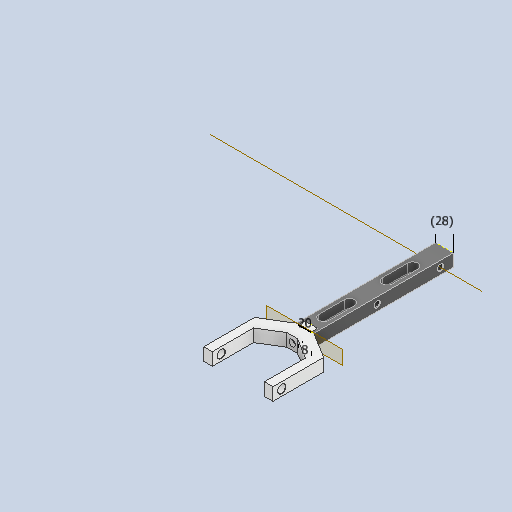
# Autodesk Inventor part: Adaptationhorizontalachse_Rillenkugellager
Saved by Autodesk Inventor 2024 (Build 280153000, 153)
## iProperties
Created: 2022-02-28
Part Number: Adaptationhorizontalachse_Rillenkugellager
Material: PBT-Kunststoff
Document SubType Name: Modeling
Designer: 123St
Density: 1.31 g/cm^3
Appearance: Glatt - Weiß
Mass: 228.778 g
Surface Area: 480.28 cm^2
Volume: 174.64 cm^3
Fixation_dist1: -20,000 mm
Fixation_dist2: -100,000 mm
Gabel_FixierungPart_Width: 28,000 mm
Author: 123St
Autodesk Inventor part; units mm, degrees
note: some values were not read from the file. Chosen so that the rebuilt part matches the saved one: direction of "Bohrung3"; direction of "Bohrung4".
sketch "Skizze1" plane through (0, 0, 0) normal (0, 1, 0) x (-1, 0, 0)
  line L0 (54.5, 104.8161) -> (54.5, 24.8161)
  line L1 (54.5, 24.8161) -> (14, 0)
  line L2 (14, 0) -> (-14, 0)
  line L3 (-14, 0) -> (-54.5, 24.8161)
  line L4 (-54.5, 24.8161) -> (-54.5, 104.8161)
  line L5 (-54.5, 104.8161) -> (-41, 104.8161)
  line L6 (-41, 104.8161) -> (-41, 40)
  line L7 (-41, 40) -> (-8.3599, 20)
  line L8 (-8.3599, 20) -> (8.3599, 20)
  line L9 (8.3599, 20) -> (41, 40)
  line L10 (41, 40) -> (41, 104.8161)
  line L11 (41, 104.8161) -> (54.5, 104.8161)
  line L12 (0, -284.9632) -> (0, 169.7793) construction
  line L13 (41, 40) -> (54.5, 40) construction
  point P0 (0, 0)
  point P1 (0, 20)
  dimension "d0" = 82
  dimension "d1" = 13.5
  dimension "d2" = 13.5
  dimension "d113" = 28
  dimension "d114" = 20
  dimension "d115" = 80
  dimension "d117" = 20
  dimension "d118" = 20
  constraints: 26 end point, 5 parallel, 5 perpendicular, 3 midpoint, 3 point on line, 2 equal length, 1 vertical
  measures "d0" distance between parallel lines of L6 L10
  measures "d1" distance between parallel lines of L10 L0
  measures "d2" distance of L4.end L5.end
  measures "d113" distance of L1.end L2.end
  measures "d114" distance between parallel lines of L8 L2
  measures "d115" distance from line of L5 L3.end
  measures "d117" distance between parallel lines of L3 L7
  measures "d118" distance from line of L8.end L13
extrude "Extrusion1" add sketch "Skizze1" along normal blind 20
sketch "Skizze2" plane through (14, 0, 0) normal (0, 0, -1) x (-1, 0, 0)
  line L0 (55, 20) -> (22.3599, 20) construction
  line L1 (0, 0) -> (28, 0)
  line L2 (28, 0) -> (28, 20)
  line L3 (28, 20) -> (0, 20)
  line L4 (0, 20) -> (0, 0)
  line L5 (14, -4) -> (14, 24) construction
  line L6 (0, 0) -> (28, 0) construction
  point P0 (14, 0)
  point P1 (14, 0)
  point P2 (14, 20)
  dimension "d75" = 28
  constraints: 8 end point, 3 midpoint, 2 parallel, 2 point on line, 1 horizontal, 1 perpendicular
  measures "d75" distance between parallel lines of L2 L4
extrude "Extrusion2" add sketch "Skizze2" along normal blind 220
ref_plane "Arbeitsebene1" through (53.5, 2, 88) normal (1, 0, 0) x (0, 0, -1)
sketch "Skizze3" plane through (54.5, 0, 104.8161) normal (1, 0, 0) x (0, 0, -1)
  line L0 (0, 10) -> (14, 10) construction
  line L1 (0, 0) -> (0, 20) construction
  circle A0 centre (14, 10) radius 6
  dimension "d44" = 14
  dimension "d87" = 12
  constraints: 2 end point, 1 centre point, 1 coincident, 1 horizontal, 1 midpoint
  measures "d44" distance of L0.start L0.end
  measures "d87" diameter of A0
extrude "Extrusion3" cut sketch "Skizze3" against normal through all
ref_plane "Arbeitsebene5" through (14, 0, -200) normal (0, 0, -1) x (-1, 0, 0)
ref_plane "Arbeitsebene6" through (14, 0, -100) normal (0, 0, -1) x (-1, 0, 0)
ref_plane "Arbeitsebene7" through (14, 0, -150) normal (0, 0, -1) x (-1, 0, 0)
sketch "Skizze13" plane through (14, 0, 104.8161) normal (1, 0, 0) x (0, 0, -1)
  line L0 (304.8161, 24) -> (304.8161, -4) construction
  line L1 (204.8161, 24) -> (204.8161, -4) construction
  line L2 (324.8161, 0) -> (324.8161, 20) construction
  line L3 (324.8161, 10) -> (204.8161, 10) construction
  point P0 (104.8161, 0)
  point P1 (304.8161, 10)
  constraints: 3 midpoint, 2 end point, 1 coincident, 1 perpendicular, 1 point on line
hole "Bohrung2" at (14, 10, -100) at (14, 10, -200) direction (-1, 0, 0) diameter 8.376 end through all thread size "M10x1.5" class "6H" standard "ISO Metric profile"
sketch "Skizze12" plane through (14, 0, -220) normal (0, 0, -1) x (-1, 0, 0)
  line L0 (28, 20) -> (0, 20) construction
  point P0 (14, 0)
  dimension "Gabel_FixierungPart_Width" = 28
  measures "Gabel_FixierungPart_Width" distance of L0.start L0.end
chamfer "Fase1" distance 0.75 angle 45 4 edges at (14, 10, -95.812) (14, 10, -195.812) (-14, 10, -195.812) (-14, 10, -95.812)
chamfer "Fase2" distance 0.5 angle 45 4 edges at (54.5, 10, 96.8161) (41, 10, 96.8161) (-54.5, 10, 96.8161) (-41, 10, 96.8161)
sketch "Skizze15" plane through (0, 20, 0) normal (0, 1, 0) x (1, 0, 0)
  line L0 (-76.3, 100) -> (76.3, 100) construction
  line L1 (0, 30) -> (0, 70) construction
  line L2 (8, 30) -> (8, 70)
  line L3 (-8, 70) -> (-8, 30)
  arc A0 (-8, 30) -> (8, 30) centre (0, 30) ccw
  arc A1 (8, 70) -> (-8, 70) centre (0, 70) ccw
  line L4 (-14, 0) -> (-14, 220) construction
  line L5 (14, 0) -> (14, 220) construction
  line L6 (-14, 100) -> (14, 100) construction
  line L7 (-14, 100) -> (14, 100) construction
  line L8 (-76.3, 200) -> (76.3, 200) construction
  line L9 (-14, 200) -> (14, 200) construction
  line L10 (0, 130) -> (0, 170) construction
  line L11 (8, 130) -> (8, 170)
  line L12 (-8, 170) -> (-8, 130)
  arc A2 (-8, 130) -> (8, 130) centre (0, 130) ccw
  arc A3 (8, 170) -> (-8, 170) centre (0, 170) ccw
  line L13 (0, 264) -> (0, -44) construction
  point P0 (0, 0)
  point P1 (0, 50)
  point P2 (0, 100)
  point P3 (0, 100)
  point P4 (0, 150)
  point P5 (0, 200)
  dimension "d124" = 0
  dimension "d125" = 100
  dimension "d126" = 50
  dimension "d127" = 40
  dimension "d130" = 0
  dimension "d131" = 0
  dimension "d133" = 40
  dimension "d134" = 100
  dimension "d135" = 50
  dimension "d156" = 16
  dimension "d157" = 16
  constraints: 22 end point, 8 point on circle, 8 point on line, 8 tangent, 5 midpoint, 4 centre point, 2 collinear, 2 horizontal, 2 parallel, 2 vertical, 1 perpendicular
  measures "d124" distance between parallel lines of L0 L6
  measures "d125" distance of point (0, 0) point (0, 100)
  measures "d126" distance of point (0, 50) point (0, 0)
  measures "d127" distance of L1.start L1.end
  measures "d130" distance between parallel lines of L0 L7
  measures "d131" distance between parallel lines of L8 L9
  measures "d133" distance of L10.start L10.end
  measures "d134" distance between parallel lines of L9 L7
  measures "d135" distance of point (0, 150) point (0, 200)
  measures "d156" distance between parallel lines of L2 L3
  measures "d157" distance between parallel lines of L11 L12
extrude "Extrusion13" cut sketch "Skizze15" against normal blind 14
ref_plane "Arbeitsebene8" through (0, 0, 0) normal (1, 0, 0) x (0, 0, -1)
ref_plane "Arbeitsebene9" through (14, 0, 0) normal (0, 0, 1) x (0, 1, 0)
split body "Trennen1" result two bodies by plane through (14, 0, 0) normal (0, 0, 1) first body at (-50, 0.5, 56.5441)
sketch "Skizze16" plane through (14, 0, 0) normal (0, 0, 1) x (0, 1, 0)
  line L0 (0, 0) -> (20, 0) construction
  line L1 (0, 0) -> (0, 28) construction
  line L2 (0, 28) -> (20, 28) construction
  line L3 (20, 28) -> (20, 0) construction
  line L4 (20, 4) -> (20, 24)
  line L5 (20, 24) -> (0, 18)
  line L6 (0, 18) -> (0, 10)
  line L7 (0, 10) -> (20, 4)
  line L8 (0, 14) -> (20, 14) construction
  point P0 (0, 14)
  point P1 (10, 14)
  dimension "d136" = 20
  dimension "d137" = 8
  constraints: 10 end point, 4 midpoint, 2 collinear, 1 horizontal, 1 parallel, 1 vertical
  measures "d136" distance of L4.end L4.start
  measures "d137" distance of L5.end L6.end
extrude "Extrusion14" add sketch "Skizze16" against normal blind 10 bodies 2
extrude "Extrusion15" cut sketch "Skizze16" against normal blind 10 bodies 3
sketch "Skizze17" plane through (-8.3599, 0, 20) normal (0, 0, 1) x (1, 0, 0)
  point P0 (8.3599, 0)
  point P1 (8.3599, 10)
hole "Bohrung3" at (0, 10, 20) direction (0, 0, -1) diameter 5.5 depth 30 counterbore diameter 10 counterbore depth 5.5 bodies 2 clearance for "Inbusschraube DIN EN ISO 4762" size "M5" standard "DIN"
sketch "Skizze18" plane through (14, 0, -10) normal (0, 0, 1) x (1, 0, 0)
  point P0 (-14, 0)
  point P1 (-14, 10)
hole "Bohrung4" at (0, 10, 0) direction (0, 0, -1) diameter 4.134 end up to surface bodies 3 thread size "M5x0.8" class "6H" standard "ISO Metric profile"
equation "\"d1\" = d2"
equation "\"d113\" = -2 * Gabel_FixationShaft_Contact_Thickness + MainAxis_Schluesselweite + 2 * ParallelMecha_Bearing_Step_Thickness - 2 * Anlaufscheibe_Ueberstand"
equation "\"d75\" = -2 * Gabel_FixationShaft_Contact_Thickness + MainAxis_Schluesselweite + 2 * ParallelMecha_Bearing_Step_Thickness - 2 * Anlaufscheibe_Ueberstand"
equation "\"ParallelMecha_Bearing_Step_Thickness\" = 6"
equation "\"Anlaufscheibe_Ueberstand\" = 0.5"
equation "\"Gabel_FixationShaft_Contact_Thickness\" = 3.5"
equation "\"MainAxis_Schluesselweite\" = 24"
